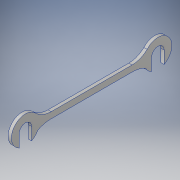
# Autodesk Inventor part: ARM LONG
Saved by Autodesk Inventor 2018 (Build 220112000, 112)
## iProperties
Created: 2018-02-28
Part Number: ARM LONG
Material: Aluminum 6061
Document SubType Name: Modeling
Designer: 238438
Density: 2.7 g/cm^3
Appearance: Aluminum - Flat
Mass: 0.0498256 g
Surface Area: 1.06895 cm^2
Volume: 0.0184539 cm^3
Author: 238438
Autodesk Inventor part; units mm, degrees
ref_plane "YZ Plane" through (0, 0, 0) normal (1, 0, 0) x (0, 1, 0)
ref_plane "XZ Plane" through (0, 0, 0) normal (0, 1, 0) x (-1, 0, 0)
ref_plane "XY Plane" through (0, 0, 0) normal (0, 0, 1) x (1, 0, 0)
sketch "Sketch1" plane through (0, 0, 0) normal (1, 0, 0) x (0, 1, 0)
  arc A0 (1.5875, 0.6096) -> (1.5875, 2.5654) centre (1.5875, 1.5875) ccw
  line L0 (1.5875, 2.5654) -> (-0.38, 2.5654)
  line L1 (1.5875, 0.6096) -> (-0.38, 0.6096)
  arc A1 (-0.38, 0.6096) -> (0.6038, -0.3771) centre (1.5875, 1.5875) ccw
  arc A2 (2.9985, -0.0967) -> (-0.38, 2.5654) centre (1.5875, 1.5875) ccw
  arc A3 (2.9985, -0.0967) -> (2.0575, -2.4657) centre (5.4835, -2.4551) ccw
  arc A4 (1.0923, -2.4605) -> (0.6038, -0.3771) centre (-3.6193, -2.4662) ccw
  line L2 (1.0923, -2.4593) -> (1.0923, -8.8093)
  line L3 (2.0575, -8.8157) -> (2.0575, -2.4657)
  arc A5 (1.5875, -20.1904) -> (1.5875, -18.2346) centre (1.5875, -19.2125) ccw
  line L4 (1.5875, -20.1904) -> (-0.38, -20.1904)
  line L5 (1.5875, -18.2346) -> (-0.38, -18.2346)
  arc A6 (0.6038, -17.2479) -> (-0.38, -18.2346) centre (1.5875, -19.2125) ccw
  arc A7 (-0.38, -20.1904) -> (2.9985, -17.5283) centre (1.5875, -19.2125) ccw
  arc A8 (2.0575, -15.1698) -> (2.9985, -17.5283) centre (5.4835, -15.1698) ccw
  arc A9 (0.6038, -17.2479) -> (1.0923, -15.1581) centre (-3.6193, -15.1587) ccw
  line L6 (1.0923, -15.1593) -> (1.0923, -8.8093)
  line L7 (2.0575, -8.8157) -> (2.0575, -15.1698)
  line L8 (2.0575, -2.4657) -> (2.0575, -15.1698)
  line L9 (1.0923, -15.1581) -> (1.0923, -2.4593)
  dimension "d11" = 1.9558
  constraints: 21 point on circle, 20 end point, 10 centre point, 4 coincident, 3 tangent, 2 horizontal, 2 parallel, 2 point on line, 1 collinear
  measures "d11" diameter of A0
extrude "Extrusion2" add sketch "Sketch1" along normal blind 0.508
body "Solid2"
